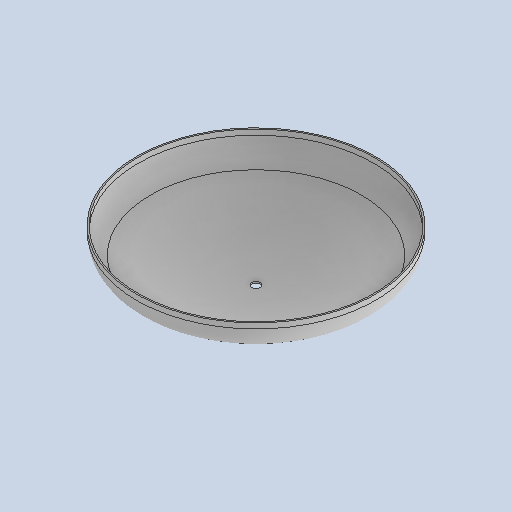
# Autodesk Inventor part: TZS 0908 dished head
Saved by Autodesk Inventor 2025 (Build 290162010, 162A)
## iProperties
Created: 2025-02-16
Part Number: TZS 0908 dished head
Material: Steel
Document SubType Name: Modeling
Designer: pokla
Density: 7.85 g/cm^3
Appearance: Default
Mass: 71183.4 g
Surface Area: 30460.9 cm^2
Volume: 9067.95 cm^3
Author: pokla
Autodesk Inventor part; units mm, degrees
ref_plane "YZ Plane" through (0, 0, 0) normal (1, 0, 0) x (0, 1, 0)
ref_plane "XZ Plane" through (0, 0, 0) normal (0, 1, 0) x (-1, 0, 0)
ref_plane "XY Plane" through (0, 0, 0) normal (0, 0, 1) x (1, 0, 0)
sketch "Sketch1" plane through (0, 0, 0) normal (0, 1, 0) x (-1, 0, 0)
  line L0 (477.5, 0) -> (477.5, -21)
  arc A0 (423.1378, -109.9786) -> (477.5, -21) centre (377.5, -21) ccw
  arc A1 (17.5, -212) -> (423.1378, -109.9786) centre (0, 715.0002) ccw
  line L1 (0, 212) -> (0, -212)
  arc A2 (17.5, -205.9989) -> (420.3995, -104.6399) centre (0, 715.0002) ccw
  arc A3 (420.3995, -104.6399) -> (471.5, -21) centre (377.5, -21) ccw
  line L2 (471.5, -21) -> (471.5, 0)
  line L3 (471.5, 0) -> (477.5, 0)
  line L4 (0, -212) -> (17.5, -212)
  line L5 (0, -205.9989) -> (17.5, -205.9989)
  line L6 (17.5, -212) -> (17.5, -205.9989)
  point P0 (0, 0)
  point P1 (0, 0)
  point P2 (0, -163.7009)
  point P3 (0, -169.7009)
  dimension "d0" = 100
  dimension "d1" = 21
  dimension "d3" = 927.1653
  dimension "d6" = 6
  dimension "d13" = 35
  dimension "d14" = 955
  dimension "d15" = 212
  constraints: 14 end point, 8 point on circle, 4 centre point, 2 horizontal, 2 parallel, 2 tangent, 2 vertical, 1 coincident, 1 horizontal alignment, 1 line through centre, 1 midpoint, 1 perpendicular, 1 point on line, 2 other
  measures "d0" radius of A0
  measures "d1" distance of L0.start L0.end
  measures "d3" radius of A1
  measures "d6" radial gap between concentric circles of A1 A2
  measures "d13" diameter of L4.end L1
  measures "d14" diameter of L0 L1
  measures "d15" distance of point (0, 0) L1.end
revolve "Revolution1" add sketch "Sketch1" angle 360 about axis through (0, 0, 212) along (0, 0, -1) contours L0 A0 A1 L6 A2 A3 L2 L3
equation "\"d0\" = tech_dishhead_small_rad"
equation "\"d1\" = tech_dishhead_edge_hight"
equation "\"d13\" = tech_dishhead_bottom_hole"
equation "\"d14\" = MAIN_filter_diam"
equation "\"d15\" = MAIN_dished_head_hight"
equation "\"tech_dishhead_small_rad\" = 100"
equation "\"tech_dishhead_edge_hight\" = 21"
equation "\"tech_dishhead_bottom_hole\" = 35"
equation "\"MAIN_filter_diam\" = 955"
equation "\"MAIN_dished_head_hight\" = 212"
body "Solid1"
